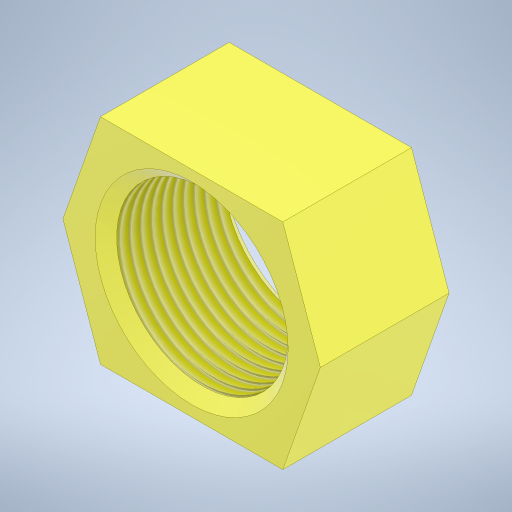
# Autodesk Inventor part: 2-HUDSON-8-35-TDR HAND PUMP M8x5 PIPE NU
Saved by Autodesk Inventor 2024.2 (Build 282272000, 272)
## iProperties
Created: 2024-11-02
Part Number: 2-HUDSON-8-35-TDR HAND PUMP M8x5 PIPE NU
Material: Genérico
Document SubType Name: Modeling
Designer: brene
Density: 1 g/cm^3
Appearance: Suave - Amarillo
Author: brene
Autodesk Inventor part; units mm, degrees
ref_plane "YZ Plane" through (0, 0, 0) normal (1, 0, 0) x (0, 1, 0)
ref_plane "XZ Plane" through (0, 0, 0) normal (0, 1, 0) x (-1, 0, 0)
ref_plane "XY Plane" through (0, 0, 0) normal (0, 0, 1) x (1, 0, 0)
sketch "Boceto1" plane through (0, 0, 0) normal (0, 0, 1) x (1, 0, 0)
  circle A0 centre (0, 0) radius 4
  line L0 (-37.8416, 0) -> (37.8416, 0) construction
  line L1 (0, 25.1226) -> (0, -25.1226) construction
  line L2 (-4.25, 5) -> (4.25, 5)
  line L3 (-4.25, -5) -> (4.25, -5)
  line L4 (-4.25, 5) -> (-6, 0)
  line L5 (-4.25, -5) -> (-6, 0)
  line L6 (4.25, 5) -> (6, 0)
  line L7 (4.25, -5) -> (6, 0)
  point P0 (0, 5)
  point P1 (0, -5)
  dimension "d0" = 8
  dimension "d1" = 8.5
  dimension "d2" = 8.5
  dimension "d3" = 5
  dimension "d4" = 5
  dimension "d5" = 6
  dimension "d6" = 6
  constraints: 16 end point, 4 midpoint, 4 point on line, 3 horizontal, 2 coincident, 1 centre point, 1 vertical
  measures "d0" diameter of A0
  measures "d1" distance of L2.start L2.end
  measures "d2" distance of L3.start L3.end
  measures "d3" distance from line of L0 L2.start
  measures "d4" distance from line of L0 L3.start
  measures "d5" distance of L6.end point (0, 0)
  measures "d6" distance of point (0, 0) L4.end
extrude "Extrusión1" add sketch "Boceto1" against normal blind 6
thread "Rosca1" size "M8x0.5" class "6H" standard "ANSI Metric M Profile" length 14
chamfer "Chaflán1" distance 0.5 angle 45 1 edges at (-4, 0, 0)
chamfer "Chaflán2" distance 0.5 angle 45 1 edges at (-4, 0, -6)
equation "\"d2\" = d1"
equation "\"d4\" = d3"
